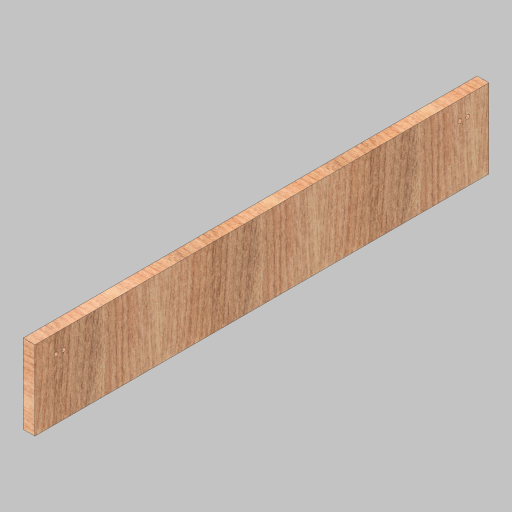
# Autodesk Inventor part: BP-002
Saved by Autodesk Inventor 2023.5 (Build 275446000, 446)
## iProperties
Created: 2025-01-26
Part Number: BP-002
Material: Wood (Birch)
Document SubType Name: Modeling
Designer: slick
Density: 0.55 g/cm^3
Appearance: Birch - Natural Polished
Author: slick
Autodesk Inventor part; units mm, degrees
ref_plane "YZ Plane" through (0, 0, 0) normal (1, 0, 0) x (0, 1, 0)
ref_plane "XZ Plane" through (0, 0, 0) normal (0, 1, 0) x (-1, 0, 0)
ref_plane "XY Plane" through (0, 0, 0) normal (0, 0, 1) x (1, 0, 0)
sketch "Sketch1" plane through (0, 0, 0) normal (1, 0, 0) x (0, 1, 0)
  line L0 (-63.5, -365.125) -> (63.5, -365.125)
  line L1 (63.5, -365.125) -> (63.5, 365.125)
  line L2 (63.5, 365.125) -> (-63.5, 365.125)
  line L3 (-63.5, 365.125) -> (-63.5, -365.125)
  line L4 (-63.5, -365.125) -> (63.5, 365.125) construction
  line L5 (63.5, -365.125) -> (-63.5, 365.125) construction
  point P0 (0, 0)
  dimension "d0" = 127
  dimension "d1" = 730.25
  constraints: 12 end point, 2 midpoint, 2 parallel, 1 horizontal, 1 perpendicular
  measures "d0" distance of L2.end L1.end
  measures "d1" distance of L0.end L1.end
extrude "Extrusion1" add sketch "Sketch1" along normal blind 19.05
sketch "Sketch2" plane through (19.05, 0, 0) normal (1, 0, 0) x (0, 0, -1)
  line L0 (-365.125, 63.5) -> (-365.125, -63.5) projected
  line L1 (365.125, 63.5) -> (-365.125, 63.5) projected
  line L2 (0, 63.5) -> (0, -57.15) construction
  point P0 (0, 0)
  point P1 (-331.0636, 33.3248)
  point P2 (-318.3636, 33.3248)
  point P3 (331.0636, 33.3248)
  point P4 (318.3636, 33.3248)
  dimension "d4" = 34.0614
  dimension "d5" = 12.7
  dimension "d6" = 30.1752
  constraints: 2 end point, 2 symmetric about line, 1 horizontal alignment, 1 midpoint, 1 vertical
  measures "d4" distance from line of L0 point (-331.064, 33.325)
  measures "d5" distance of point (-318.364, 33.325) point (-331.064, 33.325)
  measures "d6" distance from line of L1 point (-331.064, 33.325)
hole "Hole1" at (19.05, 33.3248, 331.0636) at (19.05, 33.3248, 318.3636) at (19.05, 33.3248, -331.0636) at (19.05, 33.3248, -318.3636) direction (-1, 0, 0) diameter 6.35 end through all
body "Solid1"
